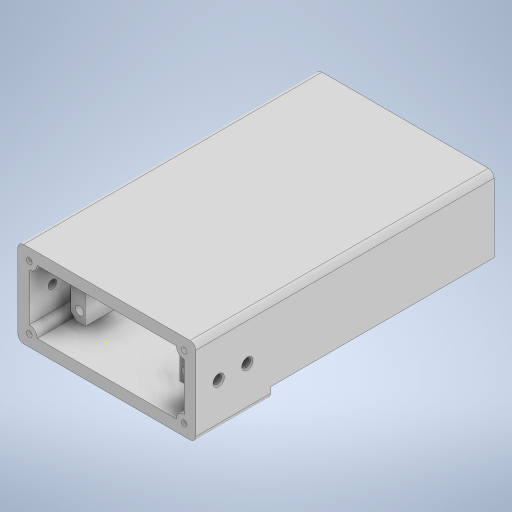
# Autodesk Inventor part: 커튼 하우징
Saved by Autodesk Inventor 2023.1 (Build 271208000, 208)
## iProperties
Created: 2022-09-03
Part Number: 커튼 하우징
Material: 일반
Document SubType Name: Modeling
Designer: fly01
Density: 1 g/cm^3
Appearance: 기본값
Author: fly01
Autodesk Inventor part; units mm, degrees
ref_plane "YZ Plane" through (0, 0, 0) normal (1, 0, 0) x (0, 1, 0)
ref_plane "XZ Plane" through (0, 0, 0) normal (0, 1, 0) x (-1, 0, 0)
ref_plane "XY Plane" through (0, 0, 0) normal (0, 0, 1) x (1, 0, 0)
sketch "스케치1" plane through (0, 0, 0) normal (0, 0, 1) x (1, 0, 0)
  line L0 (-27, -11) -> (27, -11)
  line L1 (27, -11) -> (27, 11)
  line L2 (27, 11) -> (-27, 11)
  line L3 (-27, 11) -> (-27, -11)
  line L4 (-27, -11) -> (27, 11) construction
  line L5 (27, -11) -> (-27, 11) construction
  circle A0 centre (16, 0) radius 10
  line L6 (-26, 5) -> (4, 5)
  line L7 (4, 5) -> (4, -5)
  line L8 (4, -5) -> (-26, -5)
  line L9 (-26, -5) -> (-26, 5)
  line L10 (-26, 5) -> (4, -5) construction
  line L11 (4, 5) -> (-26, -5) construction
  line L12 (-31, -15) -> (31, -15)
  line L13 (31, -15) -> (31, 15)
  line L14 (31, 15) -> (-31, 15)
  line L15 (-31, 15) -> (-31, -15)
  line L16 (27, -11) -> (31, -11)
  line L17 (-27, -11) -> (-31, -11)
  point P0 (0, 0)
  point P1 (-11, 0)
  point P2 (4, 0)
  dimension "d0" = 54
  dimension "d1" = 22
  dimension "d5" = 20
  dimension "d6" = 10
  dimension "d7" = 30
  dimension "d10" = 11
  dimension "d11" = 1
  dimension "d13" = 4
  constraints: 36 end point, 6 parallel, 5 midpoint, 4 perpendicular, 3 point on line, 2 horizontal, 2 horizontal alignment, 1 centre point, 3 other
  measures "d0" distance of L1.end L2.end
  measures "d1" distance of L0.end L1.end
  measures "d5" diameter of A0
  measures "d6" distance of L6.end L7.end
  measures "d7" distance of L7.end L8.end
  measures "d10" distance from line of L1 A0.centre
  measures "d11" distance between parallel lines of L3 L9
  measures "d13" distance between parallel lines of L3 L15
extrude "돌출1" add sketch "스케치1" against normal blind 3 contours L3 L2 L1 L0 | L17 L15 L14 L13 L16 L1 L2 L3 | A0 | L6 L7 L8 L9
extrude "돌출2" add sketch "스케치1" along normal blind 75 contours L17 L15 L14 L13 L16 L1 L2 L3
sketch "스케치2" plane through (0, 0, 0) normal (0, 0, 1) x (1, 0, 0)
  circle A0 centre (16, 0) radius 10 projected
  circle A1 centre (16, 0) radius 11
  line L0 (16, 0) -> (7.5735, -7.0707)
  line L1 (16, 0) -> (16, -11)
  line L2 (-27, -11) -> (27, -11) projected
  line L3 (16, 0) -> (24.4265, -7.0707)
  line L4 (5, 0) -> (5, 11)
  line L5 (27, 11) -> (-27, 11) projected
  line L6 (16, 11) -> (5, 11)
  line L7 (16, 11) -> (27, 11)
  line L8 (27, 11) -> (27, 0)
  line L9 (27, 11) -> (27, -11) projected
  point P0 (0, 0)
  point P1 (8.3396, -6.4279)
  point P2 (23.6604, -6.4279)
  point P3 (24.4265, -7.0707)
  point P4 (27, 0)
  dimension "d18" = 1
  dimension "d19" = 50
  constraints: 14 end point, 4 point on circle, 3 point on line, 1 centre point, 1 midpoint, 1 perpendicular, 1 symmetric about line, 1 vertical
  measures "d18" radial gap between concentric circles of A0 A1
  measures "d19" angle of L1 L0
extrude "돌출3" add sketch "스케치2" along normal blind 74 contours A0 L0 A1 L3 | L4 L5 A1 | A1 L5 L8
fillet "모깎기1" radius 0.5 4 edges at (7.5735, -7.0707, 37) (8.3396, -6.4279, 37) (23.6604, -6.4279, 37) (24.4265, -7.0707, 37)
extrude "돌출4" cut sketch "스케치2" along normal blind 3 contours A0 L0 A1 L3 | L4 L5 A1
sketch "스케치3" plane through (-27, 11, 75) normal (0, -1, 0) x (1, 0, 0)
  line L0 (3.45, -57.85) -> (28.55, -57.85) construction
  line L1 (28.55, -57.85) -> (28.55, -5.75) construction
  line L2 (28.55, -5.75) -> (3.45, -5.75) construction
  line L3 (3.45, -5.75) -> (3.45, -57.85) construction
  line L4 (3.45, -57.85) -> (28.55, -5.75) construction
  line L5 (28.55, -57.85) -> (3.45, -5.75) construction
  line L6 (0.4, -60.6) -> (31.6, -60.6) construction
  line L7 (31.6, -60.6) -> (31.6, -3) construction
  line L8 (31.6, -3) -> (0.4, -3) construction
  line L9 (0.4, -3) -> (0.4, -60.6) construction
  line L10 (0.4, -60.6) -> (31.6, -3) construction
  line L11 (31.6, -60.6) -> (0.4, -3) construction
  line L12 (32, -1) -> (0, -1) construction
  line L13 (0, -75) -> (0, 0) projected
  line L14 (0, 0) -> (54, 0) projected
  line L15 (16, -31.8) -> (18.2955, -31.8)
  line L16 (16, -31.8) -> (16, -27.2694)
  line L17 (5.95, -3.25) -> (0.95, -3.25)
  line L18 (0.95, -3.25) -> (0.95, -8.25)
  line L19 (0.95, -8.25) -> (5.95, -8.25)
  line L20 (5.95, -8.25) -> (5.95, -3.25)
  line L21 (5.95, -3.25) -> (0.95, -8.25) construction
  line L22 (0.95, -3.25) -> (5.95, -8.25) construction
  line L23 (26.05, -3.25) -> (31.05, -3.25)
  line L24 (31.05, -3.25) -> (31.05, -8.25)
  line L25 (31.05, -8.25) -> (26.05, -8.25)
  line L26 (26.05, -8.25) -> (26.05, -3.25)
  line L27 (26.05, -3.25) -> (31.05, -8.25) construction
  line L28 (31.05, -3.25) -> (26.05, -8.25) construction
  line L29 (28.55, -57.85) -> (3.45, -57.85) construction
  line L30 (5.95, -60.35) -> (0.95, -60.35)
  line L31 (0.95, -60.35) -> (0.95, -55.35)
  line L32 (0.95, -55.35) -> (5.95, -55.35)
  line L33 (5.95, -55.35) -> (5.95, -60.35)
  line L34 (5.95, -60.35) -> (0.95, -55.35) construction
  line L35 (0.95, -60.35) -> (5.95, -55.35) construction
  line L36 (31.05, -55.35) -> (26.05, -55.35)
  line L37 (26.05, -55.35) -> (26.05, -60.35)
  line L38 (31.05, -60.35) -> (31.05, -55.35)
  line L39 (31.05, -60.35) -> (26.05, -55.35) construction
  line L40 (26.05, -60.35) -> (31.05, -60.35)
  line L41 (26.05, -60.35) -> (31.05, -55.35) construction
  circle A0 centre (3.45, -5.75) radius 1
  circle A1 centre (28.55, -5.75) radius 1
  circle A2 centre (3.45, -57.85) radius 1
  circle A3 centre (28.55, -57.85) radius 1
  point P0 (27, -75)
  point P1 (16, -1)
  point P2 (16, -3)
  point P3 (16, -60.6)
  dimension "d25" = 25.1
  dimension "d26" = 52.1
  dimension "d27" = 31.2
  dimension "d28" = 57.6
  dimension "d29" = 3
  dimension "d31" = 5
  dimension "d32" = 5
  dimension "d33" = 2
  constraints: 80 end point, 16 symmetric about line, 8 midpoint, 6 parallel, 5 horizontal, 4 centre point, 3 perpendicular, 1 coincident, 1 point on line, 1 vertical, 1 vertical alignment, 3 other
  measures "d25" distance of L1.end L2.end
  measures "d26" distance of L0.end L1.end
  measures "d27" distance of L8.end L7.end
  measures "d28" distance of L7.end L6.end
  measures "d29" distance between parallel lines of L14 L8
  measures "d31" distance of L18.end L19.end
  measures "d32" distance of L19.end L17.start
  measures "d33" diameter of A0
extrude "돌출5" add sketch "스케치3" along normal blind 3
extrude "돌출6" cut sketch "스케치3" against normal blind 2 contours A0 | A1 | A2 | A3
chamfer "모따기1" distance 3 angle 45 4 edges at (-23.55, 11, 66.75) (1.55, 11, 66.75) (-23.55, 11, 14.65) (1.55, 11, 14.65)
sketch "스케치4" plane through (0, 0, -3) normal (0, 0, -1) x (-1, 0, 0)
  line L0 (25, 2) -> (11, 2)
  line L1 (11, 2) -> (11, 11)
  line L2 (11, 11) -> (25, 11)
  line L3 (25, 11) -> (25, 2)
  line L4 (25, 2) -> (11, 11) construction
  line L5 (11, 2) -> (25, 11) construction
  line L6 (31, -11) -> (31, 15) projected
  line L7 (31, 15) -> (-31, 15) projected
  point P0 (0, 0)
  point P1 (18, 6.5)
  dimension "d41" = 14
  dimension "d42" = 9
  dimension "d43" = 6
  dimension "d44" = 4
  constraints: 12 end point, 2 midpoint, 2 parallel, 1 horizontal, 1 perpendicular
  measures "d41" distance of L0.start L0.end
  measures "d42" distance of L0.end L1.end
  measures "d43" distance between parallel lines of L6 L3
  measures "d44" distance between parallel lines of L7 L2
extrude "돌출7" cut sketch "스케치4" against normal blind 14
sketch "스케치5" plane through (0, 0, 75) normal (0, 0, 1) x (1, 0, 0)
  line L0 (-31, 15) -> (31, 15)
  line L1 (31, 15) -> (31, -15)
  line L2 (31, -15) -> (-31, -15)
  line L3 (-31, -15) -> (-31, 15)
  line L4 (27, -11) -> (31, -11) projected
  point P0 (0, 0)
  dimension "d47" = 4
  constraints: 8 end point, 2 parallel, 1 horizontal, 1 perpendicular
  measures "d47" distance between parallel lines of L4 L2
extrude "돌출8" add sketch "스케치5" along normal blind 3
sketch "스케치6" plane through (0, 0, 78) normal (0, 0, 1) x (1, 0, 0)
  line L0 (-31, 15) -> (-31, -15) projected
  line L1 (-31, -15) -> (31, -15) projected
  line L2 (31, -15) -> (31, 15) projected
  line L3 (31, 15) -> (-31, 15) projected
  line L4 (-16.5, 8) -> (16.5, 8)
  line L5 (16.5, 8) -> (16.5, -8)
  line L6 (16.5, -8) -> (-16.5, -8)
  line L7 (-16.5, -8) -> (-16.5, 8)
  line L8 (-16.5, 8) -> (16.5, -8) construction
  line L9 (16.5, 8) -> (-16.5, -8) construction
  line L10 (-21.5, 8) -> (21.5, 8)
  line L11 (21.5, 8) -> (21.5, -8)
  line L12 (21.5, -8) -> (-21.5, -8)
  line L13 (-21.5, -8) -> (-21.5, 8)
  line L14 (-21.5, 8) -> (21.5, -8) construction
  line L15 (21.5, 8) -> (-21.5, -8) construction
  line L16 (-11.5, 3.5) -> (-21.5, 3.5)
  line L17 (-21.5, 3.5) -> (-21.5, -3.5)
  line L18 (-21.5, -3.5) -> (-11.5, -3.5)
  line L19 (-11.5, -3.5) -> (-11.5, 3.5)
  line L20 (-11.5, 3.5) -> (-21.5, -3.5) construction
  line L21 (-21.5, 3.5) -> (-11.5, -3.5) construction
  point P0 (0, 0)
  point P1 (-16.5, 0)
  point P2 (-16.5, 3.5)
  point P3 (-16.5, -3.5)
  dimension "d50" = 33
  dimension "d51" = 16
  dimension "d52" = 43
  dimension "d53" = 7
  constraints: 36 end point, 7 midpoint, 6 parallel, 3 horizontal, 3 perpendicular, 1 point on line
  measures "d50" distance of L4.start L4.end
  measures "d51" distance of L4.end L5.end
  measures "d52" distance of L10.start L10.end
  measures "d53" distance of L18.end L16.start
extrude "돌출9" cut sketch "스케치6" against normal blind 3 contours L16 L19 L18 L7
extrude "돌출10" add sketch "스케치6" along normal blind 14 contours L7 L16 L13 L10 | L10 L11 L12 L5 | L7 L18 L13 L16 | L7 L12 L13 L18
sketch "스케치7" plane through (0, 0, 92) normal (0, 0, 1) x (1, 0, 0)
  circle A0 centre (-18.5, 4.25) radius 1.5
  line L0 (0, 0) -> (0, 4.5353)
  line L1 (0, 0) -> (-4.0563, 0)
  circle A1 centre (-18.5, -4.25) radius 1.5
  circle A2 centre (18.5, 4.25) radius 1.5
  circle A3 centre (18.5, -4.25) radius 1.5
  dimension "d58" = 3
  dimension "d59" = 8.5
  dimension "d60" = 37
  constraints: 4 centre point, 4 end point, 3 symmetric about line, 1 horizontal, 1 vertical, 3 other
  measures "d58" diameter of A0
  measures "d59" distance of A1.centre A0.centre
  measures "d60" distance of A2.centre A0.centre
extrude "돌출11" cut sketch "스케치7" against normal blind 14
chamfer "모따기2" distance 2 angle 45 4 edges at (-21.5, -8, 85) (21.5, -8, 85) (21.5, 8, 85) (-21.5, 8, 85)
fillet "모깎기2" radius 2 10 edges at (-18, -8, 78) (-20.5, -7, 78) (-21.5, 0, 78) (18, -8, 78) (20.5, -7, 78) (21.5, 0, 78) (20.5, 7, 78) (18, 8, 78) (-20.5, 7, 78) (-18, 8, 78)
sketch "스케치8" plane through (0, 0, 78) normal (0, 0, 1) x (1, 0, 0)
  line L0 (16.5, -10) -> (16.5, 10) projected
  line L1 (20.3284, 10) -> (16.5, 10) projected
  line L2 (23.5, 6.8284) -> (20.3284, 10) projected
  line L3 (23.5, -6.8284) -> (23.5, 6.8284) projected
  line L4 (20.3284, -10) -> (23.5, -6.8284) projected
  line L5 (16.5, -10) -> (20.3284, -10) projected
  line L6 (-16.5, 10) -> (-16.5, 3.5) projected
  line L7 (-16.5, 3.5) -> (-11.5, 3.5) projected
  line L8 (-11.5, 3.5) -> (-11.5, -3.5) projected
  line L9 (-11.5, -3.5) -> (-16.5, -3.5) projected
  line L10 (-16.5, -3.5) -> (-16.5, -10) projected
  line L11 (-20.3284, -10) -> (-16.5, -10) projected
  line L12 (-23.5, -6.8284) -> (-20.3284, -10) projected
  line L13 (-23.5, 6.8284) -> (-23.5, -6.8284) projected
  line L14 (-20.3284, 10) -> (-23.5, 6.8284) projected
  line L15 (-16.5, 10) -> (-20.3284, 10) projected
  line L16 (-31, 15) -> (-31, -15) projected
  line L17 (-31, -15) -> (31, -15) projected
  line L18 (31, -15) -> (31, 15) projected
  line L19 (31, 15) -> (-31, 15) projected
  line L20 (-27, 11) -> (-27, -11)
  line L21 (-27, -11) -> (27, -11)
  line L22 (27, -11) -> (27, 11)
  line L23 (27, 11) -> (-27, 11)
  circle A0 centre (-27, 11) radius 1
  circle A1 centre (-27, 11) radius 2.75
  line L24 (0, 0) -> (-4.1541, 0)
  line L25 (0, 0) -> (0, 3.5)
  circle A2 centre (27, 11) radius 1
  circle A3 centre (27, 11) radius 2.75
  circle A4 centre (-27, -11) radius 1
  circle A5 centre (-27, -11) radius 2.75
  circle A6 centre (27, -11) radius 1
  circle A7 centre (27, -11) radius 2.75
  point P0 (-24.25, 11)
  point P1 (24.25, 11)
  point P2 (27, 8.25)
  point P3 (27, -8.25)
  point P4 (24.25, -11)
  point P5 (-24.25, -11)
  point P6 (-27, -8.25)
  point P7 (-27, 8.25)
  dimension "d68" = 2
  dimension "d69" = 5.5
  constraints: 12 end point, 8 centre point, 8 coincident, 6 symmetric about line, 1 horizontal, 1 vertical, 9 other
  measures "d68" diameter of A0
  measures "d69" diameter of A1
extrude "돌출12" add sketch "스케치8" along normal blind 23 contours L19 L18 L17 L16 | A0 L23 A1 L20 | L20 A1 L23 A0 | A5 L21 A4 L20 | L20 A4 L21 A5 | A3 L22 A2 L23 | L23 A2 L22 A3 | A7 L22 A6 L21 | L21 A6 L22 A7
sketch "스케치9" plane through (5, 11, 74) normal (0, -1, 0) x (1, 0, 0)
  line L0 (-5, -74) -> (-5, -71) construction
  circle A0 centre (-5, -71) radius 1.5
  circle A1 centre (-5, -71) radius 3
  line L1 (-32, -74) -> (22, -74) projected
  line L2 (-2, -71) -> (-2, -74)
  line L3 (-8, -71) -> (-8, -74)
  point P0 (-5, -74)
  dimension "d73" = 3
  dimension "d74" = 6
  dimension "d75" = 6
  constraints: 6 end point, 3 point on circle, 2 centre point, 2 coincident, 2 perpendicular, 2 point on line, 1 midpoint, 1 tangent, 1 vertical
  measures "d73" diameter of A0
  measures "d74" diameter of A1
  measures "d75" distance between parallel lines of L2 L3
extrude "돌출13" add sketch "스케치9" along normal blind 22
sketch "스케치10" plane through (-31, -11, -3) normal (0, -1, 0) x (1, 0, 0)
  line L0 (4, 3) -> (4, 78) projected
  line L1 (4, 3) -> (28, 3) projected
  line L2 (34, 3) -> (58, 3) projected
  line L3 (58, 3) -> (58, 78) projected
  line L4 (2.1, 78) -> (2.1, 1.1)
  line L5 (2.1, 1.1) -> (28.4, 1.1)
  line L6 (33, 1.1) -> (59.9, 1.1)
  line L7 (59.9, 1.1) -> (59.9, 78)
  line L8 (28.4, 1.1) -> (33, 1.1)
  line L9 (0, 78) -> (62, 78) projected
  arc A0 (34, 6) -> (28, 6) centre (31, 6) ccw projected
  line L10 (34, 3) -> (34, 6) projected
  circle A1 centre (31, 6) radius 1.5 projected
  line L11 (28, 6) -> (28, 3) projected
  point P0 (31, 3)
  dimension "d78" = 1.9
  dimension "d79" = 1.9
  constraints: 10 end point, 2 other
  measures "d78" distance between parallel lines of L0 L4
  measures "d79" distance between parallel lines of L2 L6
extrude "돌출14" add sketch "스케치10" along normal blind 1.4 contours L1 L11 A0 L10 L2 L3 L9 L7 L6 L8 L5 L4 L0
fillet "모깎기4" radius 2 4 edges at (-31, -15, 88) (31, -15, 88) (-31, 15, 49) (31, 15, 49)
sketch "스케치13" plane through (0, 0, 101) normal (0, 0, 1) x (1, 0, 0)
  point P0 (0, 0)
sketch "스케치14" plane through (-31, -11, -3) normal (-1, 0, 0) x (0, 0, 1)
  circle A0 centre (96, 11) radius 1.5
  circle A1 centre (86, 11) radius 1.5
  line L0 (104, 24) -> (104, -2) projected
  point P0 (3, 11)
  point P1 (104, 11)
  point P2 (104, 11)
  dimension "d84" = 3
  dimension "d85" = 3
  dimension "d86" = 10
  dimension "d87" = 8
  constraints: 2 centre point, 2 horizontal alignment, 2 midpoint
  measures "d84" diameter of A0
  measures "d85" diameter of A1
  measures "d86" distance of A0.centre A1.centre
  measures "d87" distance from line of L0 A0.centre
extrude "돌출15" cut sketch "스케치14" against normal blind 4
mirror "미러1" about plane through (0, 0, 0) normal (1, 0, 0) of "돌출15"
chamfer "모따기4" distance 0.5 angle 45 4 edges at (-31, 0, 91.5) (-31, 0, 81.5) (31, 0, 91.5) (31, 0, 81.5)
